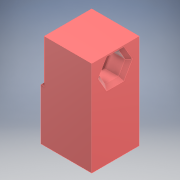
# Autodesk Inventor part: 000.001.001 - Уголок
Saved by Autodesk Inventor 2022 (Build 260153000, 153)
## iProperties
Created: 2022-02-23
Part Number: 000.001.001 - Уголок
Material: Пластик АБС
Document SubType Name: Modeling
Designer: Petrov Ivan
Density: 1.06 g/cm^3
Appearance: Гладкий — белый
Author: Petrov Ivan
Autodesk Inventor part; units mm, degrees
ref_plane "YZ Plane" through (0, 0, 0) normal (1, 0, 0) x (0, 1, 0)
ref_plane "XZ Plane" through (0, 0, 0) normal (0, 1, 0) x (-1, 0, 0)
ref_plane "XY Plane" through (0, 0, 0) normal (0, 0, 1) x (1, 0, 0)
sketch "Эскиз1" plane through (0, 0, 0) normal (0, 1, 0) x (-1, 0, 0)
  line L0 (-13.9, 13.9) -> (13.9, 13.9)
  line L1 (13.9, 13.9) -> (13.9, -13.9)
  line L2 (13.9, -13.9) -> (-13.9, -13.9)
  line L3 (-13.9, -13.9) -> (-13.9, 13.9)
  line L4 (-13.9, 13.9) -> (13.9, -13.9) construction
  line L5 (13.9, 13.9) -> (-13.9, -13.9) construction
  point P0 (0, 0)
  dimension "d0" = 27.8
  dimension "d1" = 27.8
  constraints: 12 end point, 2 midpoint, 2 parallel, 1 horizontal, 1 perpendicular
  measures "d0" distance of L1.end L2.end
  measures "d1" distance of L0.end L1.end
extrude "Выдавливание1" add sketch "Эскиз1" along normal blind 55.6
sketch "Эскиз2" plane through (0, 0, 0) normal (0, -1, 0) x (1, 0, 0)
  circle A0 centre (0.1, 0.1) radius 4 projected
  point P0 (0, 0)
extrude "Выдавливание2" cut sketch "Эскиз2" against normal blind 32
sketch "Эскиз3" plane through (-13.9, 0, -13.9) normal (-1, 0, 0) x (0, 0, 1)
  circle A0 centre (14, 46) radius 4 projected
  point P0 (13.9, 0)
extrude "Выдавливание3" cut sketch "Эскиз3" against normal through all
sketch "Эскиз4" plane through (13.9, 0, 13.9) normal (1, 0, 0) x (0, 0, -1)
  circle A0 centre (13.8, 46) radius 4 projected
  line L0 (6.0058, 46) -> (9.9029, 52.75)
  line L1 (9.9029, 52.75) -> (17.6971, 52.75)
  line L2 (17.6971, 52.75) -> (21.5942, 46)
  line L3 (21.5942, 46) -> (17.6971, 39.25)
  line L4 (17.6971, 39.25) -> (9.9029, 39.25)
  line L5 (9.9029, 39.25) -> (6.0058, 46)
  line L6 (0, 55.6) -> (27.8, 55.6) projected
  point P0 (13.9, 0)
  dimension "d8" = 13.5
  constraints: 12 end point, 1 coincident, 1 parallel, 13 other
  measures "d8" distance between parallel lines of L4 L1
extrude "Выдавливание4" cut sketch "Эскиз4" against normal blind 10
chamfer "Фаска1" distance 2 angle 45 6 edges at (13.9, 39.25, 0.1) (13.9, 42.625, -5.7457) (13.9, 49.375, -5.7457) (13.9, 52.75, 0.1) (13.9, 49.375, 5.9457) (13.9, 42.625, 5.9457)
ref_plane "РабПлоскость1" through (0.1, 22, 0.1) normal (0, -1, 0) x (1, 0, 0)
sketch "Эскиз5" plane through (0.1, 22, 0.1) normal (0, -1, 0) x (1, 0, 0)
  line L0 (-0.1, 7.9829) -> (6.9, 3.9415)
  line L1 (6.9, 3.9415) -> (6.9, -4.1415)
  line L2 (6.9, -4.1415) -> (-0.1, -8.1829)
  line L3 (-0.1, -8.1829) -> (-7.1, -4.1415)
  line L4 (-7.1, -4.1415) -> (-7.1, 3.9415)
  line L5 (-7.1, 3.9415) -> (-0.1, 7.9829)
  line L6 (-0.1, 7.9829) -> (-14, 7.9829)
  line L7 (-14, -14) -> (-14, 13.8) projected
  line L8 (-0.1, -8.1829) -> (-14, -8.1829)
  line L9 (-14, 7.9829) -> (-14, -8.1829)
  point P0 (-0.1, -0.1)
  point P1 (-0.1, -0.1)
  dimension "d15" = 14
  constraints: 18 end point, 2 point on line, 1 coincident, 1 collinear, 1 horizontal, 1 parallel, 13 other
  measures "d15" distance between parallel lines of L1 L4
extrude "Выдавливание5" cut sketch "Эскиз5" along normal mid plane 10
chamfer "Фаска2" distance 2 angle 45 4 edges at (-13.9, 27, 0) (-13.9, 22, 8.0829) (-13.9, 17, 0) (-13.9, 22, -8.0829)
sketch "Эскиз6" plane through (-13.9, 0, -13.9) normal (-1, 0, 0) x (0, 0, 1)
  line L0 (27.8, 0) -> (27.8, 55.6) projected
  line L1 (0, 0) -> (0, 55.6) projected
  line L2 (27.8, 0) -> (0, 0)
  line L3 (0, 0) -> (0, 30)
  line L4 (0, 30) -> (27.8, 30)
  line L5 (27.8, 30) -> (27.8, 0)
  line L6 (23.9829, 15) -> (23.9829, 29) projected
  line L7 (3.8171, 15) -> (23.9829, 15) projected
  line L8 (3.8171, 29) -> (3.8171, 15) projected
  line L9 (23.9829, 29) -> (3.8171, 29) projected
  point P0 (13.9, 0)
  dimension "d21" = 30
  constraints: 8 end point, 2 parallel, 1 horizontal, 1 perpendicular, 1 point on line
  measures "d21" distance of L2.end L3.end
extrude "Выдавливание6" add sketch "Эскиз6" along normal blind 2
equation "\"d1\" = d0"
equation "\"d2\" = 2 * d0"
